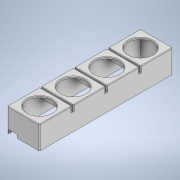
# Autodesk Inventor part: Knob_Base
Saved by Autodesk Inventor 2021 (Build 250183000, 183)
## iProperties
Created: 2020-07-22
Part Number: Knob_Base
Material: Generic
Document SubType Name: Modeling
Designer: ameli
Density: 1 g/cm^3
Appearance: Default
Author: ameli
Autodesk Inventor part; units mm, degrees
ref_plane "YZ Plane" through (0, 0, 0) normal (1, 0, 0) x (0, 1, 0)
ref_plane "XZ Plane" through (0, 0, 0) normal (0, 1, 0) x (-1, 0, 0)
ref_plane "XY Plane" through (0, 0, 0) normal (0, 0, 1) x (1, 0, 0)
sketch "Sketch1" plane through (0, 0, 0) normal (0, 1, 0) x (-1, 0, 0)
  line L0 (14.5, 59.5) -> (-14.5, 59.5)
  line L1 (-14.5, 59.5) -> (-14.5, -59.5)
  line L2 (-14.5, -59.5) -> (14.5, -59.5)
  line L3 (14.5, -59.5) -> (14.5, 59.5)
  point P0 (0, 0)
  dimension "d0" = 119
  dimension "d1" = 29
  dimension "d2" = 14.5
  dimension "d3" = 59.5
  constraints: 8 end point, 2 parallel, 1 horizontal, 1 perpendicular
  measures "d0" distance of L2.end L0.start
  measures "d1" distance of L1.end L2.end
  measures "d2" distance from line of point (0, 0) L3
  measures "d3" distance from line of point (0, 0) L2
extrude "Extrusion1" add sketch "Sketch1" along normal blind 20.5
sketch "Sketch2" plane through (0, 20.5, 0) normal (0, 1, 0) x (1, 0, 0)
  circle A0 centre (0, -45) radius 11
  circle A1 centre (0, -15) radius 11
  circle A2 centre (0, 15) radius 11
  circle A3 centre (0, 45) radius 11
  line L0 (-14.5, 59.5) -> (-14.5, -59.5) projected
  line L1 (-14.5, -59.5) -> (14.5, -59.5) projected
  line L2 (14.5, 59.5) -> (-14.5, 59.5) projected
  point P0 (0, 0)
  dimension "d9" = 22
  dimension "d10" = 22
  dimension "d11" = 22
  dimension "d12" = 22
  dimension "d13" = 14.5
  dimension "d14" = 14.5
  dimension "d15" = 14.5
  dimension "d16" = 14.5
  dimension "d17" = 14.5
  dimension "d18" = 14.5
  dimension "d19" = 44.5
  dimension "d20" = 44.5
  constraints: 4 centre point
  measures "d9" diameter of A0
  measures "d10" diameter of A1
  measures "d11" diameter of A2
  measures "d12" diameter of A3
  measures "d13" distance from line of L0 A0.centre
  measures "d14" distance from line of L0 A1.centre
  measures "d15" distance from line of L0 A2.centre
  measures "d16" distance from line of L0 A3.centre
  measures "d17" distance from line of L1 A0.centre
  measures "d18" distance from line of A3.centre L2
  measures "d19" distance from line of L1 A1.centre
  measures "d20" distance from line of L2 A2.centre
extrude "Extrusion2" cut sketch "Sketch2" against normal through all
sketch "Sketch3" plane through (0, 20.5, 0) normal (0, 1, 0) x (1, 0, 0)
  line L0 (-14.5, -30.5) -> (14.5, -30.5)
  line L1 (14.5, -30.5) -> (14.5, -29.5)
  line L2 (14.5, -29.5) -> (-14.5, -29.5)
  line L3 (-14.5, -29.5) -> (-14.5, -30.5)
  line L4 (-14.5, -0.5) -> (14.5, -0.5)
  line L5 (14.5, -0.5) -> (14.5, 0.5)
  line L6 (14.5, 0.5) -> (-14.5, 0.5)
  line L7 (-14.5, 0.5) -> (-14.5, -0.5)
  line L8 (-14.5, 29.5) -> (14.5, 29.5)
  line L9 (14.5, 29.5) -> (14.5, 30.5)
  line L10 (14.5, 30.5) -> (-14.5, 30.5)
  line L11 (-14.5, 30.5) -> (-14.5, 29.5)
  line L12 (-14.5, 59.5) -> (-14.5, -59.5) projected
  line L13 (-14.5, -59.5) -> (14.5, -59.5) projected
  point P0 (0, 0)
  dimension "d23" = 1
  dimension "d24" = 1
  dimension "d25" = 1
  dimension "d26" = 29
  dimension "d27" = 0
  dimension "d28" = 0
  dimension "d29" = 29
  dimension "d30" = 29
  dimension "d31" = 29
  dimension "d32" = 29
  dimension "d33" = 29
  constraints: 24 end point, 6 parallel, 3 horizontal, 3 perpendicular, 1 point on line
  measures "d23" distance of L2.end L0.start
  measures "d24" distance of L6.end L4.start
  measures "d25" distance of L10.end L8.start
  measures "d26" distance of L1.end L2.end
  measures "d27" distance between parallel lines of L12 L3
  measures "d28" distance between parallel lines of L12 L11
  measures "d29" distance of L4.start L4.end
  measures "d30" distance of L8.start L8.end
  measures "d31" distance between parallel lines of L13 L0
  measures "d32" distance between parallel lines of L4 L2
  measures "d33" distance between parallel lines of L8 L6
extrude "Extrusion3" cut sketch "Sketch3" against normal blind 5
shell "Shell2" thickness 1.5 removed faces 5 at (13.3333, 0, -5) at (10.9643, 6.8333, 45.8851) at (10.9643, 6.8333, 15.8851) at (10.9643, 6.8333, -14.1149) at (10.9643, 6.8333, -44.1149)
fillet "Fillet3" radius 1 16 edges at (14.5, 10.25, 59.5) (14.5, 10.25, -59.5) (-14.5, 10.25, 59.5) (-14.5, 10.25, -59.5) (14.5, 18, -30.5) (14.5, 18, -29.5) (14.5, 18, 0.5) (14.5, 18, -0.5) (14.5, 18, 30.5) (14.5, 18, 29.5) (-14.5, 18, -29.5) (-14.5, 18, -30.5) (-14.5, 18, 0.5) (-14.5, 18, -0.5) (-14.5, 18, 30.5) (-14.5, 18, 29.5)
fillet "Fillet4" radius 0.5 36 edges at (-14.2071, 20.5, -30.7929) (0, 20.5, -30.5) (14.2071, 20.5, -30.7929) (14.5, 20.5, -45) (14.2071, 20.5, -59.2071) (0, 20.5, -59.5) (-14.2071, 20.5, -59.2071) (-14.5, 20.5, -45) (-14.2071, 20.5, -0.7929) (0, 20.5, -0.5) (14.2071, 20.5, -0.7929) (14.5, 20.5, -15) (14.2071, 20.5, -29.2071) (0, 20.5, -29.5) (-14.2071, 20.5, -29.2071) (-14.5, 20.5, -15) (-14.2071, 20.5, 29.2071) (0, 20.5, 29.5) (14.2071, 20.5, 29.2071) (14.5, 20.5, 15) (14.2071, 20.5, 0.7929) (0, 20.5, 0.5) (-14.2071, 20.5, 0.7929) (-14.5, 20.5, 15) (-14.2071, 20.5, 59.2071) (0, 20.5, 59.5) (14.2071, 20.5, 59.2071) (14.5, 20.5, 45) (14.2071, 20.5, 30.7929) (0, 20.5, 30.5) (-14.2071, 20.5, 30.7929) (-14.5, 20.5, 45) (-11, 20.5, -45) (-11, 20.5, -15) (-11, 20.5, 15) (-11, 20.5, 45)
sketch "Sketch4" plane through (-13.5, 0, 59.5) normal (0, 0, 1) x (1, 0, 0)
  line L0 (0.8, 3) -> (8, 3)
  line L1 (8, 3) -> (8, 0)
  line L2 (8, 0) -> (0.8, 0)
  line L3 (0.8, 0) -> (0.8, 3)
  line L4 (0, 0) -> (27, 0) projected
  line L5 (-1, 20) -> (-1, 0) projected
  point P0 (13.5, 0)
  dimension "d39" = 7.2
  dimension "d40" = 3
  dimension "d41" = 0
  dimension "d42" = 1.8
  constraints: 8 end point, 2 parallel, 1 horizontal, 1 perpendicular
  measures "d39" distance of L0.start L0.end
  measures "d40" distance of L0.end L1.end
  measures "d41" distance between parallel lines of L4 L2
  measures "d42" distance between parallel lines of L5 L3
extrude "Extrusion4" cut sketch "Sketch4" against normal blind 2
body "Solid1"
